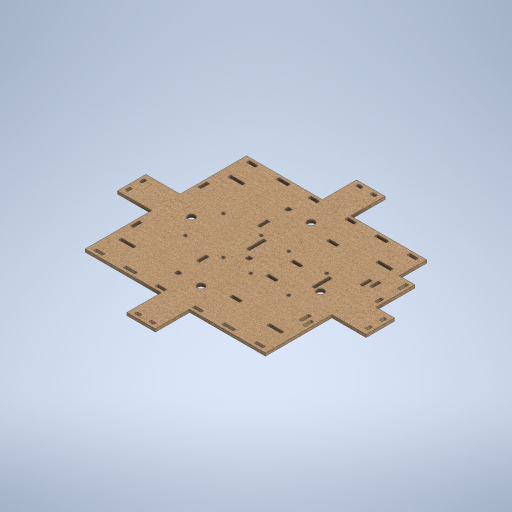
# Autodesk Inventor part: Base2
Saved by Autodesk Inventor 2024 (Build 280153000, 153)
## iProperties
Created: 2023-11-22
Part Number: Base2
Material: MDF Tablero de fibras de densidad media
Document SubType Name: Modeling
Designer: marco
Density: 0.8 g/cm^3
Appearance: Cartón - Ondulado
Author: marco
Autodesk Inventor part; units mm, degrees
ref_plane "YZ Plane" through (0, 0, 0) normal (1, 0, 0) x (0, 1, 0)
ref_plane "XZ Plane" through (0, 0, 0) normal (0, 1, 0) x (-1, 0, 0)
ref_plane "XY Plane" through (0, 0, 0) normal (0, 0, 1) x (1, 0, 0)
sketch "Boceto1" plane through (0, 0, 0) normal (0, 1, 0) x (-1, 0, 0)
  line L0 (37, -85) -> (15, -85)
  circle A0 centre (0, -58) radius 3.75
  line L1 (-15, -121) -> (15, -121)
  line L2 (15, -85) -> (15, -121)
  line L3 (-15, -82) -> (-15, -79)
  line L4 (15, -79) -> (15, -82)
  line L5 (-15, -82) -> (-24, -82)
  line L6 (-24, -82) -> (-24, -79)
  line L7 (-24, -79) -> (-15, -79)
  line L8 (15, -82) -> (24, -82)
  line L9 (24, -82) -> (24, -79)
  line L10 (24, -79) -> (15, -79)
  line L11 (15, -85) -> (95, -85)
  line L12 (95, -85) -> (95, -15)
  line L13 (95, -15) -> (131, -15)
  line L14 (-15, -121) -> (-15, -85)
  line L15 (-15, -85) -> (-95, -85)
  line L16 (-95, -85) -> (-95, -56)
  line L17 (-95, -56) -> (-111.5, -56)
  line L18 (-111.5, -56) -> (-111.5, -15)
  line L19 (-111.5, -15) -> (-131, -15)
  line L20 (-131, -15) -> (-131, 15)
  line L21 (-131, 15) -> (-95, 15)
  line L22 (-95, 15) -> (-95, 85)
  line L23 (-95, 85) -> (-15, 85)
  line L24 (-15, 85) -> (-15, 121)
  line L25 (-5, -115) -> (-5, -118)
  line L26 (-5, -118) -> (-10, -118)
  line L27 (-10, -118) -> (-10, -115)
  line L28 (-10, -115) -> (-5, -115)
  line L29 (5, -115) -> (10, -115)
  line L30 (10, -115) -> (10, -118)
  line L31 (10, -118) -> (5, -118)
  line L32 (5, -118) -> (5, -115)
  line L33 (22, -60.0916) -> (26, -60.0916)
  line L34 (26, -60.0916) -> (26, -56.0916)
  line L35 (26, -56.0916) -> (22, -56.0916)
  line L36 (22, -56.0916) -> (22, -60.0916)
  circle A1 centre (68, 0) radius 3.75
  line L37 (131, -15) -> (131, 15)
  line L38 (131, 15) -> (95, 15)
  line L39 (95, 15) -> (95, 85)
  line L40 (95, 85) -> (15, 85)
  line L41 (15, 85) -> (15, 121)
  line L42 (15, 121) -> (-15, 121)
  line L43 (125, 5) -> (125, 10)
  line L44 (125, 10) -> (128, 10)
  line L45 (128, 10) -> (128, 5)
  line L46 (128, 5) -> (125, 5)
  line L47 (128, -10) -> (125, -10)
  line L48 (125, -10) -> (125, -5)
  line L49 (125, -5) -> (128, -5)
  line L50 (128, -5) -> (128, -10)
  circle A2 centre (-14.5, -20) radius 1.5
  circle A3 centre (-14.5, 20) radius 1.5
  circle A4 centre (-54.5, 20) radius 1.5
  circle A5 centre (-54.5, -20) radius 1.5
  circle A6 centre (14.5, -20) radius 1.5
  circle A7 centre (54.5, -20) radius 1.5
  circle A8 centre (14.5, 20) radius 1.5
  circle A9 centre (54.5, 20) radius 1.5
  circle A10 centre (0, 58) radius 3.75
  circle A11 centre (-68, 0) radius 3.75
  line L51 (-89, 82) -> (-89, 79)
  line L52 (-80, 79) -> (-80, 82)
  line L53 (24, 79) -> (24, 82)
  line L54 (15, 82) -> (15, 79)
  line L55 (-89, 79) -> (-80, 79)
  line L56 (-80, 79) -> (-80, 82)
  line L57 (-80, 82) -> (-89, 82)
  line L58 (-15, 82) -> (-24, 82)
  line L59 (-24, 82) -> (-24, 79)
  line L60 (-24, 79) -> (-15, 79)
  line L61 (-15, 79) -> (-15, 82)
  line L62 (15, 79) -> (24, 79)
  line L63 (24, 79) -> (24, 82)
  line L64 (24, 82) -> (15, 82)
  line L65 (9.875, 0) -> (9.875, -18)
  line L66 (9.875, -18) -> (6.875, -18)
  line L67 (6.875, -18) -> (6.875, 0)
  line L68 (6.875, 0) -> (9.875, 0)
  line L69 (26, 60) -> (22, 60)
  line L70 (22, 60) -> (22, 56)
  line L71 (22, 56) -> (26, 56)
  line L72 (26, 56) -> (26, 60)
  line L73 (-2, 9.25) -> (2, 9.25)
  line L74 (2, 9.25) -> (2, 5.25)
  line L75 (2, 5.25) -> (-2, 5.25)
  line L76 (-2, 5.25) -> (-2, 9.25)
  line L77 (-62.125, 0) -> (-59.125, 0)
  line L78 (-59.125, 0) -> (-59.125, -18)
  line L79 (-59.125, -18) -> (-62.125, -18)
  line L80 (-62.125, -18) -> (-62.125, 0)
  line L81 (-85.5, 27) -> (-82.5, 27)
  line L82 (-82.5, 27) -> (-82.5, 37)
  line L83 (-82.5, 37) -> (-85.5, 37)
  line L84 (-85.5, 37) -> (-85.5, 27)
  line L85 (25.5, 27) -> (25.5, 37)
  line L86 (25.5, 37) -> (22.5, 37)
  line L87 (22.5, 37) -> (22.5, 27)
  line L88 (22.5, 27) -> (25.5, 27)
  line L89 (-35, 11.5) -> (-25, 11.5)
  line L90 (-25, 11.5) -> (-25, 14.5)
  line L91 (-25, 14.5) -> (-35, 14.5)
  line L92 (-35, 14.5) -> (-35, 11.5)
  line L93 (-35, -14.5) -> (-25, -14.5)
  line L94 (-25, -14.5) -> (-25, -11.5)
  line L95 (-25, -11.5) -> (-35, -11.5)
  line L96 (-35, -11.5) -> (-35, -14.5)
  line L97 (-25, 49.5) -> (-35, 49.5)
  line L98 (-35, 49.5) -> (-35, 52.5)
  line L99 (-35, 52.5) -> (-25, 52.5)
  line L100 (-25, 52.5) -> (-25, 49.5)
  line L101 (-82.5, -27) -> (-82.5, -37)
  line L102 (-82.5, -37) -> (-85.5, -37)
  line L103 (-85.5, -37) -> (-85.5, -27)
  line L104 (-85.5, -27) -> (-82.5, -27)
  line L105 (22.5, -27) -> (25.5, -27)
  line L106 (25.5, -27) -> (25.5, -37)
  line L107 (25.5, -37) -> (22.5, -37)
  line L108 (22.5, -37) -> (22.5, -27)
  line L109 (46, 82) -> (46, 79)
  line L110 (46, 79) -> (58, 79)
  line L111 (58, 79) -> (58, 82)
  line L112 (58, 82) -> (46, 82)
  line L113 (-58, 82) -> (-58, 79)
  line L114 (-58, 79) -> (-46, 79)
  line L115 (-46, 79) -> (-46, 82)
  line L116 (-46, 82) -> (-58, 82)
  line L117 (-92, -40) -> (-92, -31)
  line L118 (-92, -31) -> (-89, -31)
  line L119 (-89, -31) -> (-89, -40)
  line L120 (-89, -40) -> (-92, -40)
  line L121 (-92, 31) -> (-92, 40)
  line L122 (-92, 40) -> (-89, 40)
  line L123 (-89, 40) -> (-89, 31)
  line L124 (-89, 31) -> (-92, 31)
  line L125 (-70.5, 56) -> (-70.5, 59)
  line L126 (-70.5, 59) -> (-85.5, 59)
  line L127 (-85.5, 59) -> (-85.5, 56)
  line L128 (-85.5, 56) -> (-70.5, 56)
  line L129 (89, 79) -> (89, 82)
  line L130 (80, 82) -> (89, 82)
  line L131 (89, 82) -> (89, 79)
  line L132 (89, 79) -> (80, 79)
  line L133 (80, 79) -> (80, 82)
  line L134 (92, 31) -> (92, 40)
  line L135 (92, 40) -> (89, 40)
  line L136 (89, 40) -> (89, 31)
  line L137 (89, 31) -> (92, 31)
  line L138 (70.5, 59) -> (85.5, 59)
  line L139 (85.5, 59) -> (85.5, 56)
  line L140 (85.5, 56) -> (70.5, 56)
  line L141 (70.5, 56) -> (70.5, 59)
  line L142 (89, -79) -> (89, -82)
  line L143 (46, -79) -> (46, -82)
  line L144 (46, -82) -> (58, -82)
  line L145 (58, -82) -> (58, -79)
  line L146 (58, -79) -> (46, -79)
  line L147 (80, -79) -> (89, -79)
  line L148 (89, -79) -> (89, -82)
  line L149 (89, -82) -> (80, -82)
  line L150 (80, -82) -> (80, -79)
  line L151 (70.5, -59) -> (85.5, -59)
  line L152 (85.5, -59) -> (85.5, -56)
  line L153 (85.5, -56) -> (70.5, -56)
  line L154 (70.5, -56) -> (70.5, -59)
  line L155 (92, -40) -> (92, -31)
  line L156 (92, -31) -> (89, -31)
  line L157 (89, -31) -> (89, -40)
  line L158 (89, -40) -> (92, -40)
  line L159 (-80, -82) -> (-80, -79)
  line L160 (-89, -79) -> (-89, -82)
  line L161 (-89, -82) -> (-80, -82)
  line L162 (-80, -82) -> (-80, -79)
  line L163 (-80, -79) -> (-89, -79)
  line L164 (-35, -52.5) -> (-25, -52.5)
  line L165 (-25, -52.5) -> (-25, -49.5)
  line L166 (-25, -49.5) -> (-35, -49.5)
  line L167 (-35, -49.5) -> (-35, -52.5)
  line L168 (-46, -79) -> (-46, -82)
  line L169 (-46, -82) -> (-58, -82)
  line L170 (-58, -82) -> (-58, -79)
  line L171 (-58, -79) -> (-46, -79)
  line L172 (-85.5, -56) -> (-70.5, -56)
  line L173 (-70.5, -56) -> (-70.5, -59)
  line L174 (-70.5, -59) -> (-85.5, -59)
  line L175 (-85.5, -59) -> (-85.5, -56)
  line L176 (-108.5, -20) -> (-108.5, -26)
  line L177 (-108.5, -26) -> (-105.5, -26)
  line L178 (-105.5, -26) -> (-105.5, -20)
  line L179 (-105.5, -20) -> (-108.5, -20)
  line L180 (-108.5, -52.5) -> (-108.5, -43.5)
  line L181 (-108.5, -43.5) -> (-105.5, -43.5)
  line L182 (-105.5, -43.5) -> (-105.5, -52.5)
  line L183 (-105.5, -52.5) -> (-108.5, -52.5)
  line L184 (-128, 5) -> (-128, 10)
  line L185 (-128, 10) -> (-125, 10)
  line L186 (-125, 10) -> (-125, 5)
  line L187 (-125, 5) -> (-128, 5)
  line L188 (-125, -10) -> (-128, -10)
  line L189 (-128, -10) -> (-128, -5)
  line L190 (-128, -5) -> (-125, -5)
  line L191 (-125, -5) -> (-125, -10)
  line L192 (-10, 115) -> (-5, 115)
  line L193 (-5, 115) -> (-5, 118)
  line L194 (-5, 118) -> (-10, 118)
  line L195 (-10, 118) -> (-10, 115)
  line L196 (5, 115) -> (10, 115)
  line L197 (10, 115) -> (10, 118)
  line L198 (10, 118) -> (5, 118)
  line L199 (5, 118) -> (5, 115)
  point P0 (0, 0)
  point P1 (15, -85)
  point P2 (6.875, 0)
  constraints: 400 end point, 12 centre point
extrude "Extrusión1" add sketch "Boceto1" along normal blind 3
